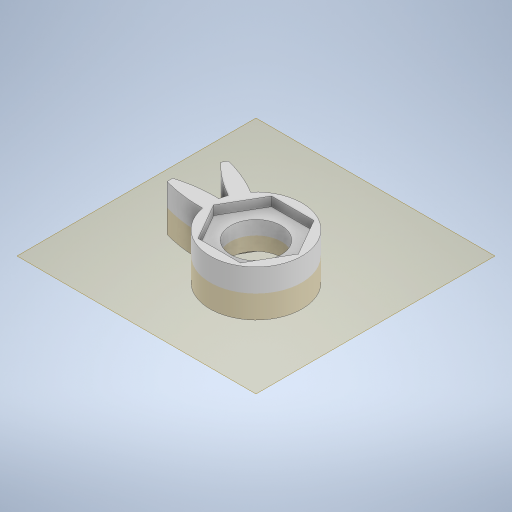
# Autodesk Inventor part: JointFixeSmallr
Saved by Autodesk Inventor 2023 (Build 270158000, 158)
## iProperties
Created: 2023-12-22
Part Number: JointFixeSmallr
Material: Generic
Document SubType Name: Modeling
Designer: Mustapha
Density: 1 g/cm^3
Appearance: Default
Author: Mustapha
Autodesk Inventor part; units mm, degrees
ref_plane "YZ Plane" through (0, 0, 0) normal (1, 0, 0) x (0, 1, 0)
ref_plane "XZ Plane" through (0, 0, 0) normal (0, 1, 0) x (-1, 0, 0)
ref_plane "XY Plane" through (0, 0, 0) normal (0, 0, 1) x (1, 0, 0)
sketch "Sketch1" plane through (0, 0, 0) normal (0, 1, 0) x (-1, 0, 0)
  circle A0 centre (0, 0) radius 5
  line L0 (5.6094, 0.8873) -> (4.9206, 0.8873)
  line L1 (4.9206, -0.8873) -> (5.6094, -0.8873)
  line L2 (13.9917, 2.0061) -> (13.9917, -2.3829)
  line L3 (9.8774, 1.3309) -> (5, 0) construction
  line L4 (5, 0) -> (9.8774, -1.3309) construction
  line L5 (9.3606, 6.8545) -> (9.3606, 0.3047)
  arc A1 (9.3606, 0.3047) -> (4.9206, 0.8873) centre (5.265, -13.6993) ccw
  line L6 (5, 0) -> (12.3774, 0)
  line L7 (9.8774, -1.3309) -> (5, 0) construction
  line L8 (9.3606, 6.8545) -> (9.3606, -0.3047)
  arc A2 (4.9206, -0.8873) -> (9.3606, -0.3047) centre (5.265, 13.6993) ccw
  arc A3 (3.8178, -3.2287) -> (7.9541, -4.9442) centre (11.4093, 9.2314) ccw
  arc A4 (8.2589, -4.4164) -> (4.705, -1.6919) centre (-2.29, -14.4964) ccw
  line L9 (11.5337, 1.2558) -> (8.2589, -4.4164)
  line L10 (11.5337, 1.2558) -> (7.9541, -4.9442)
  arc A5 (1.6919, -4.705) -> (4.4164, -8.2589) centre (14.4964, 2.29) ccw
  arc A6 (4.9442, -7.9541) -> (3.2287, -3.8178) centre (-9.2314, -11.4093) ccw
  line L11 (10.6164, -4.6793) -> (4.9442, -7.9541)
  line L12 (10.6164, -4.6793) -> (4.4164, -8.2589)
  arc A7 (-0.8873, -4.9206) -> (-0.3047, -9.3606) centre (13.6993, -5.265) ccw
  arc A8 (0.3047, -9.3606) -> (0.8873, -4.9206) centre (-13.6993, -5.265) ccw
  line L13 (6.8545, -9.3606) -> (0.3047, -9.3606)
  line L14 (6.8545, -9.3606) -> (-0.3047, -9.3606)
  arc A9 (-3.2287, -3.8178) -> (-4.9442, -7.9541) centre (9.2314, -11.4093) ccw
  arc A10 (-4.4164, -8.2589) -> (-1.6919, -4.705) centre (-14.4964, 2.29) ccw
  line L15 (1.2558, -11.5337) -> (-4.4164, -8.2589)
  line L16 (1.2558, -11.5337) -> (-4.9442, -7.9541)
  arc A11 (-4.705, -1.6919) -> (-8.2589, -4.4164) centre (2.29, -14.4964) ccw
  arc A12 (-7.9541, -4.9442) -> (-3.8178, -3.2287) centre (-11.4093, 9.2314) ccw
  line L17 (-4.6793, -10.6164) -> (-7.9541, -4.9442)
  line L18 (-4.6793, -10.6164) -> (-8.2589, -4.4164)
  arc A13 (-4.9206, 0.8873) -> (-9.3606, 0.3047) centre (-5.265, -13.6993) ccw
  arc A14 (-9.3606, -0.3047) -> (-4.9206, -0.8873) centre (-5.265, 13.6993) ccw
  line L19 (-9.3606, -6.8545) -> (-9.3606, -0.3047)
  line L20 (-9.3606, -6.8545) -> (-9.3606, 0.3047)
  arc A15 (-3.8178, 3.2287) -> (-7.9541, 4.9442) centre (-11.4093, -9.2314) ccw
  arc A16 (-8.2589, 4.4164) -> (-4.705, 1.6919) centre (2.29, 14.4964) ccw
  line L21 (-11.5337, -1.2558) -> (-8.2589, 4.4164)
  line L22 (-11.5337, -1.2558) -> (-7.9541, 4.9442)
  arc A17 (-1.6919, 4.705) -> (-4.4164, 8.2589) centre (-14.4964, -2.29) ccw
  arc A18 (-4.9442, 7.9541) -> (-3.2287, 3.8178) centre (9.2314, 11.4093) ccw
  line L23 (-10.6164, 4.6793) -> (-4.9442, 7.9541)
  line L24 (-10.6164, 4.6793) -> (-4.4164, 8.2589)
  arc A19 (0.8873, 4.9206) -> (0.3047, 9.3606) centre (-13.6993, 5.265) ccw
  arc A20 (-0.3047, 9.3606) -> (-0.8873, 4.9206) centre (13.6993, 5.265) ccw
  line L25 (-6.8545, 9.3606) -> (-0.3047, 9.3606)
  line L26 (-6.8545, 9.3606) -> (0.3047, 9.3606)
  arc A21 (3.2287, 3.8178) -> (4.9442, 7.9541) centre (-9.2314, 11.4093) ccw
  arc A22 (4.4164, 8.2589) -> (1.6919, 4.705) centre (14.4964, -2.29) ccw
  line L27 (-1.2558, 11.5337) -> (4.4164, 8.2589)
  line L28 (-1.2558, 11.5337) -> (4.9442, 7.9541)
  arc A23 (4.705, 1.6919) -> (8.2589, 4.4164) centre (-2.29, 14.4964) ccw
  arc A24 (7.9541, 4.9442) -> (3.8178, 3.2287) centre (11.4093, -9.2314) ccw
  line L29 (4.6793, 10.6164) -> (7.9541, 4.9442)
  line L30 (4.6793, 10.6164) -> (8.2589, 4.4164)
  line L31 (4.9752, -1.8432) -> (4.9752, -0.155)
  line L32 (4.9752, 0.155) -> (4.9752, 1.8432)
  line L33 (0.1623, -0.03) -> (0.1623, 0.0204)
  circle A25 centre (0, 0) radius 2.75
  point P0 (13.1202, -5.2586)
  point P1 (4.4143, -3.5731)
  point P2 (5.3016, -2.0363)
  point P3 (8.7332, -11.1141)
  point P4 (2.0363, -5.3016)
  point P5 (3.5731, -4.4143)
  point P6 (2.0061, -13.9917)
  point P7 (-0.8873, -5.6094)
  point P8 (0.8873, -5.6094)
  point P9 (-5.2586, -13.1202)
  point P10 (-3.5731, -4.4143)
  point P11 (-2.0363, -5.3016)
  point P12 (-11.1141, -8.7332)
  point P13 (-5.3016, -2.0363)
  point P14 (-4.4143, -3.5731)
  point P15 (-13.9917, -2.0061)
  point P16 (-5.6094, 0.8873)
  point P17 (-5.6094, -0.8873)
  point P18 (-13.1202, 5.2586)
  point P19 (-4.4143, 3.5731)
  point P20 (-5.3016, 2.0363)
  point P21 (-8.7332, 11.1141)
  point P22 (-2.0363, 5.3016)
  point P23 (-3.5731, 4.4143)
  point P24 (-2.0061, 13.9917)
  point P25 (0.8873, 5.6094)
  point P26 (-0.8873, 5.6094)
  point P27 (5.2586, 13.1202)
  point P28 (3.5731, 4.4143)
  point P29 (2.0363, 5.3016)
  point P30 (11.1141, 8.7332)
  point P31 (5.3016, 2.0363)
  point P32 (4.4143, 3.5731)
  point P33 (4.705, -1.6919)
  point P34 (4.9206, -0.8873)
  point P35 (4.705, 1.6919)
  point P36 (3.8178, 3.2287)
  point P37 (3.2287, 3.8178)
  point P38 (1.6919, 4.705)
  point P39 (0.8873, 4.9206)
  point P40 (-0.8873, 4.9206)
  point P41 (-1.6919, 4.705)
  point P42 (-3.2287, 3.8178)
  point P43 (-3.8178, 3.2287)
  point P44 (-4.705, 1.6919)
  point P45 (-4.9206, 0.8873)
  point P46 (-4.9206, -0.8873)
  point P47 (-4.705, -1.6919)
  point P48 (-3.8178, -3.2287)
  point P49 (-3.2287, -3.8178)
  point P50 (-1.6919, -4.705)
  point P51 (-0.8873, -4.9206)
  point P52 (0.8873, -4.9206)
  point P53 (1.6919, -4.705)
  point P54 (3.2287, -3.8178)
  point P55 (3.8178, -3.2287)
  point P56 (9.3606, 0.3047)
  point P57 (7.9541, 4.9442)
  point P58 (4.4164, 8.2589)
  point P59 (-0.3047, 9.3606)
  point P60 (-8.2589, 4.4164)
  point P61 (-9.3606, -0.3047)
  point P62 (-4.4164, -8.2589)
  point P63 (0.3047, -9.3606)
  point P64 (4.9442, -7.9541)
  point P65 (8.2589, -4.4164)
  point P66 (4.9206, -0.8873)
  dimension "d0" = 10
  dimension "d3" = 360
  dimension "d5" = 5.5
  constraints: 91 point on circle, 70 end point, 25 centre point, 4 parallel, 3 perpendicular, 3 symmetric about line, 2 coincident, 1 horizontal, 1 vertical, 174 other
  measures "d5" diameter of A25
extrude "Extrusion1" add sketch "Sketch1" along normal blind 5 contours A0 | L0 L32 A0 | L32 L0 A1 L8 L6 A0 | L6 L8 A2 L1 L31 A0 | L31 L1 A0 | A4 L10 A3 A0
sketch "Sketch2" plane through (0, 5, 0) normal (0, 1, 0) x (1, 0, 0)
  line L0 (-2.3094, 4) -> (2.3094, 4)
  line L1 (2.3094, 4) -> (4.6188, 0)
  line L2 (4.6188, 0) -> (2.3094, -4)
  line L3 (2.3094, -4) -> (-2.3094, -4)
  line L4 (-2.3094, -4) -> (-4.6188, 0)
  line L5 (-4.6188, 0) -> (-2.3094, 4)
  line L6 (0, 0) -> (-6.3613, 0)
  dimension "d8" = 8
  constraints: 14 end point, 1 coincident, 1 horizontal, 1 parallel, 13 other
  measures "d8" distance between parallel lines of L3 L0
extrude "Extrusion2" cut sketch "Sketch2" against normal blind 1
ref_plane "Work Plane1" through (0, 2.5, 0) normal (0, 1, 0) x (1, 0, 0)
mirror "Mirror1" about plane through (0, 2.5, 0) normal (0, 1, 0) of "Extrusion2"
body "Solid1"
